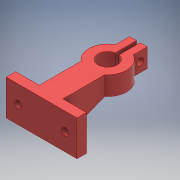
# Autodesk Inventor part: Kamera_uchwyt
Saved by Autodesk Inventor 2017 (Build 210142000, 142)
## iProperties
Created: 2018-08-13
Part Number: Kamera_uchwyt
Material: Tworzywo sztuczne PET
Document SubType Name: Modeling
Designer: Wojciech
Density: 1.541 g/cm^3
Appearance: Gładki - czerwony
Mass: 7.77531 g
Surface Area: 30.2256 cm^2
Volume: 5.04562 cm^3
Author: Wojciech
Autodesk Inventor part; units mm, degrees
ref_plane "YZ Plane" through (0, 0, 0) normal (1, 0, 0) x (0, 1, 0)
ref_plane "XZ Plane" through (0, 0, 0) normal (0, 1, 0) x (-1, 0, 0)
ref_plane "XY Plane" through (0, 0, 0) normal (0, 0, 1) x (1, 0, 0)
sketch "Szkic1" plane through (0, 0, 0) normal (0, 0, 1) x (1, 0, 0)
  line L0 (-15, -2) -> (15, -2)
  line L1 (15, -2) -> (15, 2)
  line L2 (15, 2) -> (5, 2)
  line L3 (-15, 2) -> (-15, -2)
  line L4 (-15, -2) -> (15, 2) construction
  line L5 (15, -2) -> (-15, 2) construction
  line L6 (-5, 2) -> (-0.75, 2)
  line L7 (5, 2) -> (5, 19.755)
  line L8 (5, 22) -> (-5, 22)
  line L9 (-5, 22) -> (-5, 2)
  line L10 (-0.75, 28.2995) -> (0.75, 28.2995)
  line L11 (0.75, 28.2995) -> (0.75, 33.9648)
  line L12 (0.75, 35.6626) -> (-0.75, 35.6626)
  line L13 (-0.75, 35.6626) -> (-0.75, 33.9648)
  line L14 (-0.75, 28.2995) -> (0.75, 35.6626) construction
  line L15 (0.75, 28.2995) -> (-0.75, 35.6626) construction
  line L16 (-0.75, 33.9648) -> (-0.75, 28.2995)
  arc A0 (5, 19.755) -> (0.75, 33.9648) centre (0, 26) ccw
  arc A1 (0.9, 22) -> (0.75, 30.0308) centre (0, 26) ccw
  arc A2 (-0.75, 30.0308) -> (0.9, 22) centre (0, 26) ccw
  arc A3 (-0.75, 33.9648) -> (-5, 19.755) centre (0, 26) ccw
  line L17 (0.75, 33.9648) -> (0.75, 35.6626)
  arc A4 (-5, 19.755) -> (2.749, 18.4871) centre (0, 26) ccw
  arc A5 (2.749, 18.4871) -> (5, 19.755) centre (0, 26) ccw
  line L18 (5, 19.755) -> (5, 22)
  line L19 (5, 2) -> (-15, 2)
  line L20 (-0.75, 2) -> (5, 2)
  point P0 (0, 0)
  point P1 (0, 31.981)
  dimension "d0" = 30
  dimension "d1" = 4
  dimension "d2" = 10
  dimension "d3" = 20
  dimension "d4" = 5
  dimension "d6" = 4
  dimension "d7" = 5
  dimension "d9" = 1.5
  dimension "d10" = 7.3631
  dimension "d11" = 31.981
  dimension "d12" = 5
  dimension "d13" = 8
  dimension "d14" = 4.1
  constraints: 42 end point, 12 parallel, 12 point on circle, 7 perpendicular, 7 point on line, 6 centre point, 5 midpoint, 4 horizontal, 1 coincident
  measures "d0" distance of L3.start L1.end
  measures "d1" distance of L1.end L0.end
  measures "d2" distance of L8.end L8.start
  measures "d3" distance of L8.start L2.end
  measures "d4" distance from line of point (0, 0) L9
  measures "d6" distance from line of L8 A0.centre
  measures "d7" distance from line of L9 A0.centre
  measures "d9" distance of L12.end L12.start
  measures "d10" distance of L10.end L12.start
  measures "d11" distance of point (0, 0) point (0, 31.981)
  measures "d12" distance from line of L9 point (0, 31.981)
  measures "d13" radius of A3
  measures "d14" radius of A2
extrude "Wyciągnięcie proste1" add sketch "Szkic1" against normal blind 8 contours L3 L19 L6 L2 L1 L0 | L9 A4 A5 L7 L19 L6 | A3 L16 A2 L8 L9 | L9 L8 A2 L18 A5 A4 | L18 L8 A1 L11 A0
sketch "Szkic2" plane through (0, 0, -8) normal (0, 0, -1) x (-1, 0, 0)
  line L0 (-15, 2) -> (15, 2)
  line L1 (15, 2) -> (15, -2)
  line L2 (15, -2) -> (-15, -2)
  line L3 (-15, -2) -> (-15, 2)
  point P0 (0, 0)
  constraints: 8 end point, 2 parallel, 1 horizontal, 1 perpendicular
extrude "Wyciągnięcie proste2" add sketch "Szkic2" along normal blind 7
sketch "Szkic3" plane through (-0.75, 30.0308, 0) normal (1, 0, 0) x (0, 0, -1)
  line L0 (0, 3.9339) -> (0, 0) projected
  line L1 (0, 0) -> (8, 0)
  line L2 (8, 0) -> (8, 9)
  line L3 (8, 9) -> (0, 9)
  line L4 (0, 9) -> (0, 0)
  point P0 (0, -30.0308)
  dimension "d19" = 8
  dimension "d20" = 9
  constraints: 8 end point, 2 parallel, 1 horizontal, 1 perpendicular
  measures "d19" distance of L3.end L2.end
  measures "d20" distance of L2.end L1.end
extrude "Wyciągnięcie proste3" add sketch "Szkic3" against normal blind 3
sketch "Szkic4" plane through (-3.75, 30.0308, 0) normal (-1, 0, 0) x (0, 0, 1)
  line L0 (0, 9) -> (-8, 9) projected
  line L1 (0, 3.0358) -> (0, 9) projected
  point P0 (0, -30.0308)
  point P1 (-4, 6)
  dimension "d23" = 3
  dimension "d24" = 4
  measures "d23" distance from line of L0 point (-4, 6)
  measures "d24" distance from line of L1 point (-4, 6)
hole "Otwór1" at (-3.75, 36.0308, -4) direction (1, 0, 0) diameter 3 depth 8 tip angle 118
mirror "Odbij1" about plane through (0, 0, 0) normal (1, 0, 0) of "Wyciągnięcie proste3", "Otwór1"
sketch "Szkic5" plane through (0, 0, -8) normal (0, 0, -1) x (-1, 0, 0)
  arc A0 (-3.75, 33.0666) -> (-5, 19.755) centre (0, 26) ccw projected
  line L0 (5, 2) -> (15, 2) projected
  line L1 (-5, 19.755) -> (5, 19.755)
  line L2 (5, 19.755) -> (5, 2)
  line L3 (5, 2) -> (-5, 2)
  line L4 (-5, 2) -> (-5, 19.755)
  point P0 (0, 0)
  constraints: 8 end point, 2 parallel, 1 horizontal, 1 perpendicular
extrude "Wyciągnięcie proste4" add sketch "Szkic5" along normal blind 7
sketch "Szkic7" plane through (-5, 2, 0) normal (-1, 0, 0) x (0, 0, 1)
  line L0 (0, 17.755) -> (-8, 17.755) projected
  line L1 (-15, -4) -> (-15, 0) projected
  line L2 (-8, 17.755) -> (-15, 0)
  line L3 (-15, 17.755) -> (-15, 0) projected
  line L4 (-15, 0) -> (-15, 17.755)
  line L5 (-8, 17.755) -> (-15, 17.755) projected
  line L6 (-15, 17.755) -> (-8, 17.755)
  point P0 (0, -2)
  constraints: 6 end point, 2 collinear
extrude "Wyciągnięcie proste5" cut sketch "Szkic7" against normal through all
sketch "Szkic8" plane through (-15, 2, 0) normal (0, 1, 0) x (1, 0, 0)
  line L0 (0, 0) -> (0, 15) projected
  line L1 (0, 15) -> (10, 15) projected
  line L2 (15, 0) -> (15, 15) construction
  point P0 (5, 7.5)
  point P1 (25, 7.5)
  dimension "d36" = 5
  dimension "d37" = 7.5
  constraints: 2 end point, 1 symmetric about line, 1 vertical
  measures "d36" distance from line of L0 point (5, 7.5)
  measures "d37" distance from line of L1 point (5, 7.5)
hole "Otwór2" at (-10, 2, -7.5) at (10, 2, -7.5) direction (0, -1, 0) diameter 3 depth 8 tip angle 118
